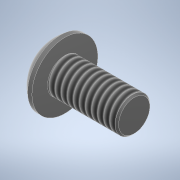
# Autodesk Inventor part: M4 x 8 mm BHCS
Saved by Autodesk Inventor 2022 (Build 260153000, 153)
## iProperties
Created: 2022-03-20
Part Number: M4 x 8 mm BHCS
Material: Generic
Document SubType Name: Modeling
Designer: Nick
Density: 1 g/cm^3
Appearance: Smooth - Black
Author: Nick
Autodesk Inventor part; units mm, degrees
ref_plane "YZ Plane" through (0, 0, 0) normal (1, 0, 0) x (0, 1, 0)
ref_plane "XZ Plane" through (0, 0, 0) normal (0, 1, 0) x (-1, 0, 0)
ref_plane "XY Plane" through (0, 0, 0) normal (0, 0, 1) x (1, 0, 0)
sketch "Sketch1" plane through (0, 0, 0) normal (0, 0, 1) x (1, 0, 0)
  line L0 (0, 0) -> (0, 1.5)
  line L1 (2.2, 3.8) -> (2.2, 2)
  line L2 (2.2, 2) -> (10.2, 2)
  line L3 (10.2, 2) -> (10.2, 0)
  line L4 (10.2, 0) -> (0, 0)
  line L5 (2.2, 3.8) -> (1.7, 3.8)
  arc A0 (1.7, 3.8) -> (0, 1.5) centre (4.0624, 0.2756) ccw
  dimension "d0" = 2.2
  dimension "d1" = 8
  dimension "d2" = 3.8
  dimension "d4" = 0.5
  dimension "d5" = 2
  dimension "d7" = 1.5
  constraints: 12 end point, 3 vertical, 2 point on circle, 1 centre point, 1 horizontal, 1 parallel, 1 perpendicular
  measures "d0" distance between parallel lines of L1 L0
  measures "d1" distance of L1.end L2.end
  measures "d2" distance between parallel lines of L4 L5
  measures "d4" distance of L1.start L5.end
  measures "d5" distance between parallel lines of L2 L4
  measures "d7" distance of L0.start L0.end
revolve "Revolution1" add sketch "Sketch1" angle 360 about axis through (10.2, 0, 0) along (-1, 0, 0)
sketch "Sketch2" plane through (0, 0, 0) normal (-1, 0, 0) x (0, 0, 1)
  line L0 (-1.25, -0.7217) -> (-1.25, 0.7217)
  line L1 (-1.25, 0.7217) -> (0, 1.4434)
  line L2 (0, 1.4434) -> (1.25, 0.7217)
  line L3 (1.25, 0.7217) -> (1.25, -0.7217)
  line L4 (1.25, -0.7217) -> (0, -1.4434)
  line L5 (0, -1.4434) -> (-1.25, -0.7217)
  point P0 (0, 0)
  point P1 (0, 0)
  dimension "d8" = 2.5
  constraints: 12 end point, 1 coincident, 1 vertical, 13 other
  measures "d8" distance between parallel lines of L3 L0
extrude "Extrusion1" cut sketch "Sketch2" against normal blind 1.3
chamfer "Chamfer1" distance 0.2 angle 45 1 edges at (10.2, -2, 0)
thread "Thread1" size "M4x0.7" class "6g" standard "ANSI Metric M Profile" full length
body "Solid1"
